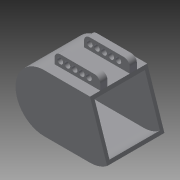
# Autodesk Inventor part: Scoop_001
Saved by Autodesk Inventor 2015 (Build 190159000, 159)
## iProperties
Created: 2016-04-07
Part Number: Scoop_001
Material: Generic
Document SubType Name: Modeling
Designer: Judson
Density: 1 g/cm^3
Appearance: Default
Author: Judson
Autodesk Inventor part; units mm, degrees
ref_plane "YZ Plane" through (0, 0, 0) normal (1, 0, 0) x (0, 1, 0)
ref_plane "XZ Plane" through (0, 0, 0) normal (0, 1, 0) x (-1, 0, 0)
ref_plane "XY Plane" through (0, 0, 0) normal (0, 0, 1) x (1, 0, 0)
sketch "Sketch1" plane through (0, 0, 0) normal (0, 0, 1) x (1, 0, 0)
  arc A0 (-50.8, 31.75) -> (-50.8, -31.75) centre (-50.8, 0) ccw
  line L0 (-50.8, 31.75) -> (0, 31.75)
  line L1 (0, -31.75) -> (-50.8, -31.75)
  arc A1 (0, -31.75) -> (0, 31.75) centre (0, 0) ccw
  constraints: 4 end point, 4 point on circle, 2 centre point, 2 tangent, 1 coincident, 1 parallel
extrude "Extrusion1" add sketch "Sketch1" against normal blind 63.5
ref_plane "Work Plane1" through (0, 0, -31.75) normal (0, 0, 1) x (1, 0, 0)
sketch "Sketch2" plane through (0, 0, -31.75) normal (0, 0, 1) x (1, 0, 0)
  arc A0 (-50.8, 31.75) -> (-50.8, -31.75) centre (-50.8, 0) ccw projected
  line L0 (-50.8, 31.75) -> (0, 31.75) projected
  arc A1 (0, -31.75) -> (0, 31.75) centre (0, 0) ccw projected
  line L1 (0, -31.75) -> (-50.8, -31.75) projected
  arc A2 (-50.8, 28.1437) -> (-50.8, -28.1437) centre (-50.8, 0) ccw
  line L2 (-50.8, 28.1437) -> (0, 28.1437)
  arc A3 (0, -28.1437) -> (0, 28.1437) centre (0, 0) ccw
  line L3 (0, -28.1437) -> (-50.8, -28.1437)
  constraints: 4 end point, 4 point on circle, 2 centre point, 3 other
extrude "Extrusion2" cut sketch "Sketch2" along normal mid plane 55.88 contours L2 A3 L3 A2
sketch "Sketch3" plane through (0, 0, 0) normal (0, 0, 1) x (1, 0, 0)
  circle A0 centre (0, 0) radius 31.75
  line L0 (0, 31.75) -> (19.0425, -25.4056)
  dimension "d7" = 63.5
  constraints: 2 end point, 2 point on circle, 1 centre point, 1 coincident
  measures "d7" diameter of A0
extrude "Extrusion3" cut sketch "Sketch3" against normal blind 63.5 contours A0 L0 picked at (8.7025, 12.4328)
sketch "Sketch4" plane through (-50.8, 31.75, 0) normal (0, 1, 0) x (1, 0, 0)
  line L0 (50.8, 0) -> (0, 0) projected
  line L1 (50.8, 0) -> (50.8, 63.5) projected
  line L2 (0, 63.5) -> (50.8, 63.5) projected
  line L3 (0, 0) -> (0, 63.5) projected
  line L4 (0, 31.75) -> (50.8, 31.75)
  line L5 (0, 0) -> (0, 63.5) projected
  line L6 (50.8, 0) -> (50.8, 63.5) projected
  line L7 (0, 11.43) -> (50.8, 11.43)
  line L8 (50.8, 11.43) -> (50.8, 52.07)
  line L9 (50.8, 52.07) -> (0, 52.07)
  line L10 (0, 52.07) -> (0, 11.43)
  line L11 (0, 19.3675) -> (50.8, 19.3675)
  line L12 (0, 44.1325) -> (50.8, 44.1325)
  dimension "d10" = 31.75
  dimension "d11" = 20.32
  dimension "d12" = 40.64
  dimension "d13" = 7.9375
  dimension "d14" = 7.9375
  constraints: 14 end point, 6 point on line, 3 perpendicular, 2 horizontal, 2 midpoint, 2 parallel
  measures "d10" distance between parallel lines of L0 L4
  measures "d11" distance between parallel lines of L9 L4
  measures "d12" distance of L9.end L7.start
  measures "d13" distance between parallel lines of L7 L11
  measures "d14" distance between parallel lines of L9 L12
extrude "Extrusion4" add sketch "Sketch4" along normal blind 12.7 contours L7 L3 L11 L1 | L12 L3 L9 L1
sketch "Sketch5" plane through (-50.8, 31.75, -11.43) normal (0, 0, 1) x (1, 0, 0)
  line L0 (50.8, 0) -> (0, 0) projected
  line L1 (50.8, 0) -> (50.8, 12.7) projected
  line L2 (0, 12.7) -> (50.8, 12.7) projected
  line L3 (0, 0) -> (0, 12.7) projected
  circle A0 centre (6.35, 6.35) radius 6.35
  circle A1 centre (44.45, 6.35) radius 6.35
  line L4 (6.35, 12.7) -> (44.45, 12.7)
  line L5 (44.45, 0) -> (6.35, 0)
  line L6 (6.35, 6.35) -> (0, 6.35)
  line L7 (44.45, 6.35) -> (50.8, 6.35)
  point P0 (50.8, -31.75)
  constraints: 8 end point, 6 point on circle, 6 tangent, 4 point on line, 2 centre point, 2 midpoint
extrude "Extrusion5" cut sketch "Sketch5" against normal blind 63.5 contours A1 L2 L1 | L3 L2 A0
sketch "Sketch6" plane through (-50.8, 31.75, -11.43) normal (0, 0, 1) x (1, 0, 0)
  arc A0 (6.35, 12.7) -> (0, 6.35) centre (6.35, 6.35) ccw projected
  line L0 (0, 0) -> (0, 6.35) projected
  line L1 (50.8, 0) -> (0, 0) projected
  line L2 (50.8, 0) -> (50.8, 6.35) projected
  arc A1 (50.8, 6.35) -> (44.45, 12.7) centre (44.45, 6.35) ccw projected
  line L3 (6.35, 12.7) -> (44.45, 12.7) projected
  circle A2 centre (6.35, 6.35) radius 3.175
  line L4 (6.35, 6.35) -> (44.45, 6.35)
  circle A3 centre (14.2875, 6.35) radius 3.175
  circle A4 centre (22.225, 6.35) radius 3.175
  circle A5 centre (30.1625, 6.35) radius 3.175
  circle A6 centre (38.1, 6.35) radius 3.175
  point P0 (50.8, -31.75)
  dimension "d19" = 6.35
  dimension "d22" = 7.9375
  constraints: 5 centre point, 2 end point, 2 horizontal, 1 coincident, 8 other
  measures "d19" diameter of A2
  measures "d22" distance of L4.start A3.centre
extrude "Extrusion6" cut sketch "Sketch6" against normal blind 63.5 contours A2 | A3 L4 | L4 A3 | A4 L4 | L4 A4 | A5 L4 | L4 A5 | A6 L4 | L4 A6
body "Solid1"
